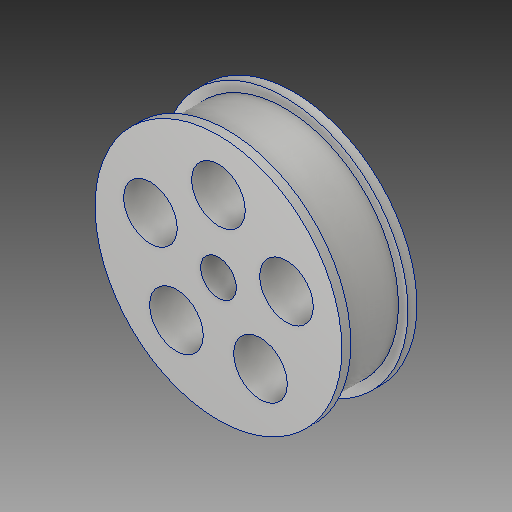
# Autodesk Inventor part: HTD 5M 60
Saved by Autodesk Inventor 2019.4 (Build 234330000, 330)
## iProperties
Created: 2020-01-22
Part Number: HTD 5M 60
Material: Aluminum 6061
Document SubType Name: Modeling
Designer: Mark
Mass: 133.43 g
Surface Area: 165.586 cm^2
Volume: 49.4185 cm^3
Density: 2.7 g/cm^3
Appearance: Aluminum - Flat
Author: Mark
Autodesk Inventor part; units mm, degrees
ref_plane "YZ Plane" through (0, 0, 0) normal (1, 0, 0) x (0, 1, 0)
ref_plane "XZ Plane" through (0, 0, 0) normal (0, 1, 0) x (-1, 0, 0)
ref_plane "XY Plane" through (0, 0, 0) normal (0, 0, 1) x (1, 0, 0)
sketch "Sketch1" plane through (0, 0, 0) normal (0, 0, 1) x (1, 0, 0)
  circle A0 centre (0, 0) radius 31.83
  dimension "d0" = 63.66
  constraints: 1 centre point, 1 coincident
  measures "d0" diameter of A0
extrude "Extrusion1" add sketch "Sketch1" along normal blind 16
sketch "Sketch2" plane through (0, 0, 16) normal (0, 0, 1) x (1, 0, 0)
  circle A0 centre (0, 0) radius 34.5
  dimension "d3" = 69
  constraints: 1 centre point, 1 coincident
  measures "d3" diameter of A0
extrude "Extrusion2" add sketch "Sketch2" along normal blind 2.5
sketch "Sketch3" plane through (0, 0, 0) normal (0, 0, -1) x (-1, 0, 0)
  circle A0 centre (0, 0) radius 34.5
  dimension "d6" = 69
  constraints: 1 centre point, 1 coincident
  measures "d6" diameter of A0
extrude "Extrusion3" add sketch "Sketch3" along normal blind 2.5
sketch "Sketch4" plane through (0, 0, -2.5) normal (0, 0, -1) x (-1, 0, 0)
  circle A0 centre (0, 0) radius 5
  circle A1 centre (0, 20) radius 7.5
  circle A2 centre (-19.0211, 6.1803) radius 7.5
  circle A3 centre (-11.7557, -16.1803) radius 7.5
  circle A4 centre (11.7557, -16.1803) radius 7.5
  circle A5 centre (19.0211, 6.1803) radius 7.5
  dimension "d9" = 10
  dimension "d10" = 15
  dimension "d11" = 20
  dimension "d14" = 360
  constraints: 6 centre point, 1 coincident, 11 other
  measures "d9" diameter of A0
  measures "d10" diameter of A1
  measures "d11" distance of A0.centre A1.centre
extrude "Extrusion4" cut sketch "Sketch4" against normal through all
body "Solid1"
